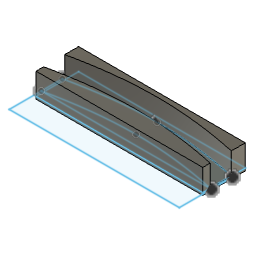
baby-bjorn v5 (Autodesk Fusion 360 design; units mm, degrees)
Autodesk Fusion 360 part; units mm, degrees
sketch "arc-thing" plane through (0, 0, 0) normal (0, 0, 1) x (1, 0, 0)
  line L0 (-66.5, 0) -> (66.5, 0)
  line L1 (66.5, 0) -> (66.5, -25)
  line L2 (66.5, -25) -> (-66.5, -25)
  line L3 (-66.5, -25) -> (-66.5, 0)
  spline S0 degree 5 poles (-66.5, 0) (-63.84, 0.5825) (-58.52, 1.6967) (-50.54, 3.2153) (-39.9, 4.9298) (-26.6, 6.5208) (-13.3, 7.5102) (0, 7.8489) (13.3, 7.5102) (26.6, 6.5208) (39.9, 4.9298) (50.54, 3.2153) (58.52, 1.6967) (63.84, 0.5825) (66.5, 0) knots 0 0 0 0 0 0 0.1 0.2 0.3 0.4 0.5 0.6 0.7 0.8 0.9 1 1 1 1 1 1
  spline S1 degree 5 poles (-66.5, 16.5) (-63.84, 17.0825) (-58.52, 18.1967) (-50.54, 19.7153) (-39.9, 21.4298) (-26.6, 23.0208) (-13.3, 24.0102) (0, 24.3489) (13.3, 24.0102) (26.6, 23.0208) (39.9, 21.4298) (50.54, 19.7153) (58.52, 18.1967) (63.84, 17.0825) (66.5, 16.5) knots 0 0 0 0 0 0 0.1 0.2 0.3 0.4 0.5 0.6 0.7 0.8 0.9 1 1 1 1 1 1
  line L4 (-66.5, 16.5) -> (-66.5, 0)
  line L5 (66.5, 16.5) -> (66.5, 0)
  line L6 (-64.9521, 27.6947) -> (65.4182, 27.6947)
  line L7 (65.4182, 27.6947) -> (65.4182, -5.6058)
  line L8 (65.4182, -5.6058) -> (-64.9521, -5.6058)
  line L9 (-64.9521, -5.6058) -> (-64.9521, 27.6947)
  point P0 (0, 7.68)
  point P1 (0, 24.18)
  dimension "d3" = 133
  dimension "d4" = 7.68
  dimension "d5" = 133
  constraint horizontal L0
  constraint vertical L1
  constraint horizontal L2
  constraint vertical L3
  constraint perpendicular L0 L4
  constraint perpendicular L0 L5
  constraint horizontal L6
  constraint vertical L7
  constraint horizontal L8
  constraint vertical L9
  measures "d3" distance of L0.start L0.end
  measures "d4" distance of L0 P0
  measures "d5" distance of S1.end S1.start
extrude "Extrude1" add sketch "arc-thing" against normal blind 2 contours L0 S0 L7 L9 | L0 L7 L8 L9 | S0 S1 L7 L9 | S1 L6 L7 L9
extrude "Extrude2" add sketch "arc-thing" along normal blind 17 contours L0 S0 L7 L9 | L0 L7 L8 L9 | S1 L6 L7 L9
equation "arc_w = 133 mm"
equation "arc_h = 7.68 mm"
equation "d3 = arc_w"
equation "d4 = arc_h"
equation "d5 = arc_w"
